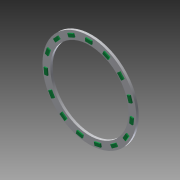
# Autodesk Inventor part: AE60-G15
Saved by Autodesk Inventor 2016 SP1 (Build 200210100, 210)
## iProperties
Category: Electrical
Company: Autodesk Inc.
Created: 2015-12-04
Part Number: AE60-G15
Material: Polypropylene
Document SubType Name: Modeling
Designer: Autodesk Inc.
Density: 0.899 g/cm^3
Appearance: White
Catalog Web Link: https://www.superbrightleds.com/moreinfo/led-accent-lighting/led-angel-eye-headlight-accent-lights/49/
Vendor: SuperBrightLEDs
Author: Autodesk Inc.
Autodesk Inventor part; units mm, degrees
ref_plane "YZ Plane" through (0, 0, 0) normal (1, 0, 0) x (0, 1, 0)
ref_plane "XZ Plane" through (0, 0, 0) normal (0, 1, 0) x (-1, 0, 0)
ref_plane "XY Plane" through (0, 0, 0) normal (0, 0, 1) x (1, 0, 0)
sketch "Sketch1" plane through (0, 0, 0) normal (0, 1, 0) x (-1, 0, 0)
  circle A0 centre (0, 0) radius 30
  circle A1 centre (0, 0) radius 25
  dimension "d0" = 60
  dimension "d1" = 50
  constraints: 2 centre point, 2 coincident
  measures "d0" diameter of A0
  measures "d1" diameter of A1
extrude "Extrusion1" add sketch "Sketch1" against normal blind 1.5
sketch "Sketch2" plane through (0, -1.5, 0) normal (0, -1, 0) x (1, 0, 0)
  line L0 (-2, 28.5) -> (2, 28.5)
  line L1 (2, 28.5) -> (2, 26.5)
  line L2 (2, 26.5) -> (-2, 26.5)
  line L3 (-2, 26.5) -> (-2, 28.5)
  point P0 (0, 0)
  point P1 (0, 28.5)
  dimension "d4" = 2
  dimension "d5" = 26.5
  dimension "d6" = 4
  constraints: 8 end point, 2 parallel, 1 horizontal, 1 midpoint, 1 perpendicular, 1 vertical alignment
  measures "d4" distance of L0.end L1.end
  measures "d5" distance from line of L2 point (0, 0)
  measures "d6" distance of L0.start L0.end
extrude "Extrusion2" add sketch "Sketch2" along normal blind 0.75
pattern_circular "Circular Pattern1" count 15 over 360 about axis through (0, -10, 0) along (0, 1, 0) of "Extrusion2"
body "Solid1"
